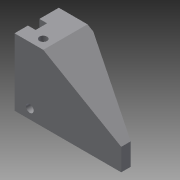
# Autodesk Inventor part: HW 2 Part 3
Saved by Autodesk Inventor 2015 (Build 190159000, 159)
## iProperties
Created: 2016-01-24
Part Number: HW 2 Part 3
Material: Generic
Document SubType Name: Modeling
Designer: Melissa
Density: 1 g/cm^3
Appearance: Default
Author: Melissa
Autodesk Inventor part; units mm, degrees
ref_plane "YZ Plane" through (0, 0, 0) normal (1, 0, 0) x (0, 1, 0)
ref_plane "XZ Plane" through (0, 0, 0) normal (0, 1, 0) x (-1, 0, 0)
ref_plane "XY Plane" through (0, 0, 0) normal (0, 0, 1) x (1, 0, 0)
sketch "Sketch1" plane through (0, 0, 0) normal (0, 0, 1) x (1, 0, 0)
  line L0 (0, 0) -> (0, 35)
  line L1 (0, 35) -> (20, 35)
  line L2 (20, 35) -> (20, 65)
  line L3 (20, 65) -> (0, 65)
  line L4 (0, 65) -> (0, 115.5325)
  line L5 (0, 115.5325) -> (90, 115.5325)
  line L6 (90, 115.5325) -> (278.4804, 25)
  line L7 (278.4804, 25) -> (278.4804, 0)
  line L8 (278.4804, 0) -> (0, 0)
  circle A0 centre (50, 25) radius 10
  dimension "d0" = 35
  dimension "d1" = 20
  dimension "d2" = 30
  dimension "d3" = 20
  dimension "d4" = 90
  dimension "d5" = 20
  dimension "d6" = 25
  dimension "d7" = 50
  dimension "d23" = 25
  constraints: 18 end point, 4 perpendicular, 2 point on line, 1 centre point, 1 parallel, 1 vertical
  measures "d0" distance of L0.start L0.end
  measures "d1" distance of L0.end L1.end
  measures "d2" distance of L1.end L2.end
  measures "d3" distance of L2.end L3.end
  measures "d4" distance of L4.end L5.end
  measures "d5" diameter of A0
  measures "d6" distance from line of L8 A0.centre
  measures "d7" distance from line of L0 A0.centre
  measures "d23" distance of L6.end L7.end
extrude "Extrusion1" add sketch "Sketch1" along normal blind 175
sketch "Sketch2" plane through (0, 115.5325, 0) normal (0, 1, 0) x (1, 0, 0)
  circle A0 centre (40, -25) radius 10
  line L0 (0, 0) -> (90, 0) projected
  line L1 (0, 0) -> (0, -175) projected
  dimension "d10" = 20
  dimension "d11" = 25
  dimension "d12" = 40
  constraints: 1 centre point
  measures "d10" diameter of A0
  measures "d11" distance from line of L0 A0.centre
  measures "d12" distance from line of A0.centre L1
extrude "Extrusion2" cut sketch "Sketch2" against normal through all
sketch "Sketch3" plane through (0, 115.5325, 0) normal (0, 1, 0) x (1, 0, 0)
  line L0 (0, -50) -> (195.2781, -50)
  line L1 (0, 0) -> (90, 0) projected
  line L2 (0, 0) -> (0, -175) projected
  line L3 (0, -125) -> (195.2781, -125)
  line L4 (195.2781, -125) -> (195.2781, -50)
  line L5 (0, -125) -> (0, -50)
  dimension "d15" = 50
  dimension "d16" = 75
  constraints: 8 end point, 3 perpendicular, 1 horizontal, 1 point on line
  measures "d15" distance between parallel lines of L1 L0
  measures "d16" distance between parallel lines of L0 L3
extrude "Extrusion3" cut sketch "Sketch3" against normal blind 25
sketch "Sketch4" plane through (0, 115.5325, 175) normal (0, 1, 0) x (1, 0, 0)
  line L0 (0, 0) -> (278.4804, 0) projected
  line L1 (75, 0) -> (320.0389, 141.4733)
  line L2 (320.0389, 141.4733) -> (320.0389, 0)
  line L3 (320.0389, 0) -> (75, 0)
  point P0 (0, 175)
  dimension "d19" = 75
  dimension "d20" = 30
  constraints: 6 end point, 3 point on line, 1 perpendicular
  measures "d19" distance of L1.start L0.start
  measures "d20" angle of L1 L0
extrude "Extrusion4" cut sketch "Sketch4" against normal through all
body "Solid1"
